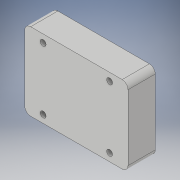
# Autodesk Inventor part: LockBooster
Saved by Autodesk Inventor 2019 (Build 230136000, 136)
## iProperties
Created: 2019-07-03
Part Number: LockBooster
Material: Generic
Document SubType Name: Modeling
Designer: garretthagen21
Density: 1 g/cm^3
Appearance: Default
Author: garretthagen21
Autodesk Inventor part; units mm, degrees
ref_plane "YZ Plane" through (0, 0, 0) normal (1, 0, 0) x (0, 1, 0)
ref_plane "XZ Plane" through (0, 0, 0) normal (0, 1, 0) x (-1, 0, 0)
ref_plane "XY Plane" through (0, 0, 0) normal (0, 0, 1) x (1, 0, 0)
sketch "Sketch1" plane through (0, 0, 0) normal (0, 0, 1) x (1, 0, 0)
  line L0 (-49.5074, 41.7962) -> (6.3726, 41.7962)
  line L1 (6.3726, 41.7962) -> (6.3726, -0.1138)
  line L2 (6.3726, -0.1138) -> (-49.5074, -0.1138)
  line L3 (-49.5074, -0.1138) -> (-49.5074, 41.7962)
  point P0 (0, 0)
  dimension "d0" = 55.88
  dimension "d1" = 41.91
  constraints: 8 end point, 2 parallel, 1 horizontal, 1 perpendicular
  measures "d0" distance of L1.end L2.end
  measures "d1" distance of L0.end L1.end
extrude "Extrusion1" add sketch "Sketch1" along normal blind 14.732
sketch "Sketch2" plane through (0, 0, 14.732) normal (0, 0, 1) x (1, 0, 0)
  line L0 (-49.5074, 41.7962) -> (-49.5074, -0.1138) projected
  line L1 (6.3726, 41.7962) -> (-49.5074, 41.7962) projected
  line L2 (6.3726, -0.1138) -> (6.3726, 41.7962) projected
  line L3 (-49.5074, -0.1138) -> (6.3726, -0.1138) projected
  point P0 (0, 0)
  point P1 (-39.5506, 37.6052)
  point P2 (-3.5842, 37.6052)
  point P3 (-3.5842, 4.0772)
  point P4 (-39.5506, 4.0772)
  dimension "d4" = 9.9568
  dimension "d5" = 4.191
  dimension "d6" = 9.9568
  dimension "d7" = 4.191
  measures "d4" distance from line of point (-39.551, 37.605) L0
  measures "d5" distance from line of point (-39.551, 37.605) L1
  measures "d6" distance from line of point (-3.584, 37.605) L2
  measures "d7" distance from line of point (-3.584, 4.077) L3
hole "Hole1" at (-39.5506, 37.6052, 14.732) at (-3.5842, 37.6052, 14.732) at (-3.5842, 4.0772, 14.732) at (-39.5506, 4.0772, 14.732) direction (0, 0, -1) diameter 3.175 end through all
fillet "Fillet1" radius 3.175 4 edges at (-49.5074, 41.7962, 7.366) (6.3726, 41.7962, 7.366) (6.3726, -0.1138, 7.366) (-49.5074, -0.1138, 7.366)
body "Solid1"
